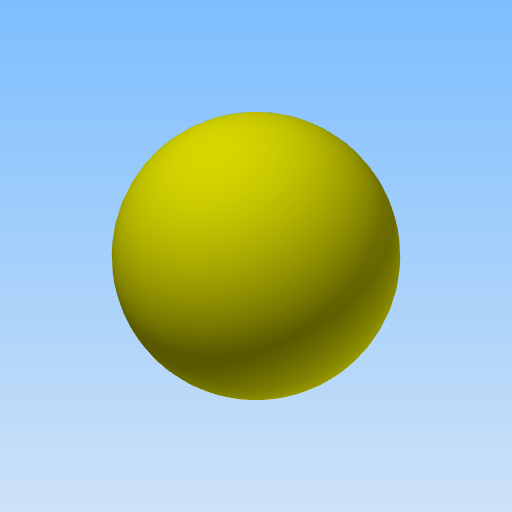
# Autodesk Inventor part: 61813-2RS1_PART3
Saved by Autodesk Inventor 2020.2 (Build 242310000, 310)
## iProperties
Created: 2020-03-01
Part Number: 61813-2RS1_PART3
Material: Allgemein
Catalog Web Link: www.cadenas.de
Description: -Deep groove ball bearings
Vendor: SKF
Document SubType Name: Modeling
Designer: psadmin
Manufacturer: SKF
Mass: 0.0898019 g
Surface Area: 0.969783 cm^2
Volume: 0.0898019 cm^3
Density: 1 g/cm^3
Appearance: PSOLRGB-192-192-192
Category: PARTsolutions
Company: SKF
PSOL_IDENT_0: {$CADENAS_DATA\23d-libs\skf\bearings_units_and_housings\ball_bearings\deep_groove_ball_bearings\bb1_
PSOL_IDENT_1: 001_101.prj},198 {VTYP=3D},{NB=61813-2RS1_PART3},{LINA=61813-2RS1_PART3},{NN=BB1_001_101_PART3},{NOP
PSOL_IDENT_2: RJ=TRUE},{DATE=19.12.2019 14:34:47},{GEOMDATE=18.12.2019 13:53:11},{VERSION=},{LINEID=7250},{WBVAR=}
PSOL_IDENT_3: ,{WBNUMERIC=}  {NB=61813-2RS1_PART3},{LINA=61813-2RS1_PART3},{KT=DUMMY},{PRODUCTID=1010271813},{DESI
PSOL_IDENT_4: GNATION=61813-2RS1},{DD=65.000},{D=85.000},{B=10.000},{C=0.000},{DD1=71.40},{DD2=0.00},{D1=0.00},{D2=
PSOL_IDENT_5: 80.50},{D3=0.000},{D4=0.000},{HH=MIN},{BB=0.000},{FF=0.00},{R0MAX=MIN},{R0=MIN},{R12=0.60},{PITCH=75
PSOL_IDENT_6: .00},{DW=5.556},{DDAMIN=68.200},{DDAMAX=71.500},{DDBMIN=MIN},{DDBMAX=MIN},{DBMIN=MIN},{DAMAX=81.800}
PSOL_IDENT_7: ,{BBAMIN=MIN},{CAMAX=MIN},{RAMAX=0.600},{LOAD1=12.400},{LOAD2=12.700},{LOAD3=0.540},{SPEED1=MIN},{SP
PSOL_IDENT_8: EED2=4500},{KR=0.015},{F0=17.000},{Z=23},{II=1},{MASS=0.130},{BEARING=61813-2RS1},{RING=},{HELP=3.13
PSOL_IDENT_9: 9},{HELP2=2.250},{DD1ALG=35.700},{YALG=35.700},{PITCH1=75.000},{DW1=5.556},{YALG1=39.361},{HALG1=3.1
PSOL_IDENT_10: 39},{SH=35.700},{CU=0.889},{DESIGN=dgbb2rs},{HALG=3.2},{B1=0},{SHIELDHELP=2}
NT: Deep groove ball bearings
NB: 61813-2RS1_PART3
NBSYN: $DESIGNATION._PART3
LINA: 61813-2RS1_PART3
SUPPLIER: SKF
ARTICLENO: 61813-2RS1_PART3
BOMINFO: 61813-2RS1_PART3
CREATOR: CADENAS GmbH
Title: 61813-2RS1_PART3
Author: Cadenas PARTsolutions
Comments: Deep groove ball bearings
Autodesk Inventor part; units mm, degrees
ref_plane "YZ Plane" through (0, 0, 0) normal (1, 0, 0) x (0, 1, 0)
ref_plane "XZ Plane" through (0, 0, 0) normal (0, 1, 0) x (-1, 0, 0)
ref_plane "XY Plane" through (0, 0, 0) normal (0, 0, 1) x (1, 0, 0)
sketch "Sketch_6" plane through (0, 0, 0) normal (0, 0, 1) x (1, 0, 0)
  line L0 (7.778, 37.5) -> (2.222, 37.5)
  arc A0 (7.778, 37.5) -> (2.222, 37.5) centre (5, 37.5) ccw
  line L1 (7.778, 37.5) -> (2.222, 37.5)
  dimension "d0" = 360
  constraints: 4 end point, 2 point on circle, 1 centre point
revolve "Revolution1" add sketch "Sketch_6" angle 360 about axis through (7.778, 37.5, 0) along (1, 0, 0)
body "Solid1"
